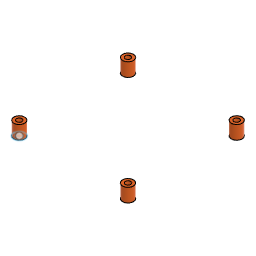
Standoff pcb (Autodesk Fusion 360 design; units mm, degrees)
Autodesk Fusion 360 part; units mm, degrees
sketch "sketch 398" plane through (0, 0, 82) normal (0, 0, 1) x (-1, 0, 0)
  circle A0 centre (-140, 40) radius 1.95
  circle A1 centre (-140, 40) radius 3.95
extrude "Extrude1" add sketch "sketch 398" along normal blind 10 makes body 1
copy_body "CopyPasteBodies1" bodies 1 makes body 2
move_body "Move1" bodies 2 to x (1, 0, 0) y (0, 1, 0) z (0, 0, 1) at (0, 80, 0)
copy_body "CopyPasteBodies2" bodies 2 1 makes body 3 makes body 4
move_body "Move2" bodies 3 4 to x (1, 0, 0) y (0, 1, 0) z (0, 0, 1) at (80, 0, 0)
